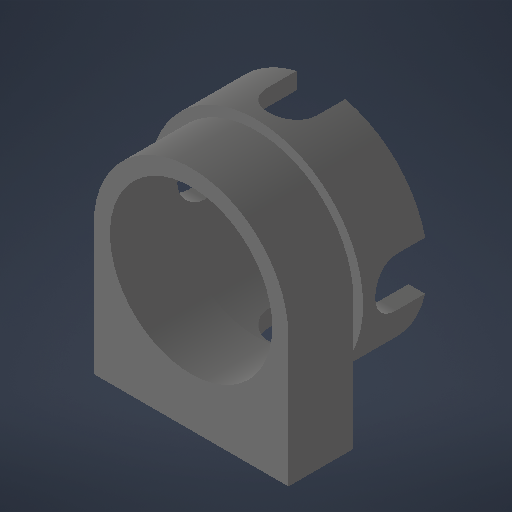
# Autodesk Inventor part: Adafruit_1528_4699_ND_House_01
Saved by Autodesk Inventor 2026.2 (Build 302298000, 298)
## iProperties
Created: 2026-02-02
Part Number: Adafruit_1528_4699_ND_House_01
Material: Generic
Document SubType Name: Modeling
Designer: vckot
Density: 1 g/cm^3
Appearance: Gray
Author: vckot
Autodesk Inventor part; units mm, degrees
ref_plane "YZ Plane" through (0, 0, 0) normal (1, 0, 0) x (0, 1, 0)
ref_plane "XY Plane" through (0, 0, 0) normal (0, 0, 1) x (1, 0, 0)
sketch "Sketch2" plane through (0, 0, 0) normal (0, 0, 1) x (1, 0, 0)
  circle A0 centre (0, 0) radius 14
  circle A1 centre (0, 0) radius 12.5
  circle A2 centre (0, 0) radius 16.5
  circle A3 centre (0, 0) radius 15
  dimension "d0" = 28
  dimension "d1" = 25
  dimension "d2" = 33
  dimension "d3" = 30
  constraints: 4 centre point, 4 coincident
  measures "d0" diameter of A0
  measures "d1" diameter of A1
  measures "d2" diameter of A2
  measures "d3" diameter of A3
extrude "Extrusion1" add sketch "Sketch2" against normal blind 10 contours A2 | A3
extrude "Extrusion2" add sketch "Sketch2" along normal blind 10 contours A0 | A3
ref_plane "Work Plane1" through (0, -20, 0) normal (0, 1, 0) x (-1, 0, 0)
sketch "Sketch3" plane through (0, -20, 0) normal (0, 1, 0) x (-1, 0, 0)
  line L0 (15, 10) -> (-15, 10) projected
  line L1 (-15, 0) -> (15, 0) projected
  line L2 (-26, 10) -> (-26, 0)
  line L3 (26, 10) -> (26, 0)
  line L4 (15, 0) -> (15, 10)
  line L5 (16.5, 0) -> (-16.5, 0) projected
  line L6 (-15, 0) -> (-16.5, 0)
  line L7 (-16.5, 0) -> (-16.5, 10)
  line L8 (-16.5, 10) -> (-15, 10)
  line L9 (16.5, 0) -> (16.5, 10)
  line L10 (16.5, 10) -> (15, 10)
  line L11 (-26, 0) -> (-16.5, 0)
  line L12 (-26, 10) -> (-16.5, 10)
  line L13 (16.5, 10) -> (26, 10)
  line L14 (-15, 0) -> (-15, 10)
  dimension "d9" = 11
  dimension "d10" = 11
  dimension "d11" = 10
  dimension "d36" = 33
  constraints: 24 end point, 3 equal length, 3 perpendicular, 2 horizontal, 2 vertical
  measures "d9" distance of L8.end L2.start
  measures "d10" distance of L3.end L4.start
  measures "d11" distance of L3.start L3.end
  measures "d36" distance between parallel lines of L9 L7
extrude "Extrusion3" add sketch "Sketch3" along normal blind 20 contours L4 L1 L14 L0
extrude "Extrusion4" [suppressed]
extrude "Extrusion5" cut sketch "Sketch2" along normal through all contours A1
sketch "Sketch4" plane through (0, -10, 0) normal (0, 1, 0) x (1, 0, 0)
  line L0 (26, -10) -> (26, 0) projected
  line L1 (15, -10) -> (26, -10) projected
  line L2 (-26, -10) -> (-15, -10) projected
  line L3 (-26, 0) -> (-26, -10) projected
  point P0 (0, 0)
  point P1 (20.5, -4.5)
  point P2 (-21, -5)
  dimension "d18" = 5.5
  dimension "d19" = 5.5
  dimension "d20" = 5
  dimension "d21" = 5
  measures "d18" distance from line of L0 point (20.5, -4.5)
  measures "d19" distance from line of L1 point (20.5, -4.5)
  measures "d20" distance from line of L2 point (-21, -5)
  measures "d21" distance from line of L3 point (-21, -5)
hole "Hole1" [suppressed]
ref_plane "Work Plane2" through (0, 16.5, 0) normal (0, -1, 0) x (1, 0, 0)
sketch "Sketch5" plane through (0, 16.5, 0) normal (0, -1, 0) x (1, 0, 0)
  line L0 (-16.5, -10) -> (16.5, -10) projected
  line L1 (-3.75, -10) -> (3.75, -10)
  line L2 (3.75, -10) -> (3.75, -5.625)
  line L3 (3.75, -5.625) -> (-3.75, -5.625)
  line L4 (-3.75, -5.625) -> (-3.75, -10)
  arc A0 (3.75, -5.625) -> (-3.75, -5.625) centre (0, -5.625) ccw
  line L5 (15, 0) -> (-15, 0) projected
  circle A1 centre (0, -5.625) radius 2.125 projected
  point P0 (0, 0)
  point P1 (0, 0)
  point P2 (-33, 0)
  point P3 (-33, 0)
  dimension "d29" = 3.75
  constraints: 8 end point, 2 midpoint, 2 parallel, 2 point on circle, 1 centre point, 1 horizontal, 1 perpendicular, 1 point on line, 1 vertical alignment
  measures "d29" radius of A0
extrude "Extrusion6" cut sketch "Sketch5" along normal blind 10
pattern_circular "Circular Pattern1" count 4 over 360 about axis through (0, 0, 0) along (0, 0, -1) of "Extrusion6"
equation "\"d18\" = 0.5 * d9"
equation "\"d19\" = 0.5 * d9"
equation "\"d20\" = 0.5 * d11"
equation "\"d21\" = 0.5 * d11"
body "Solid1"
